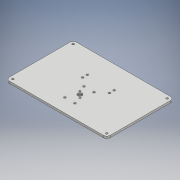
# Autodesk Inventor part: SheetPot
Saved by Autodesk Inventor 2018 (Build 220112000, 112)
## iProperties
Created: 2019-06-03
Part Number: SheetPot
Material: Generic
Document SubType Name: Modeling
Designer: aal_9
Density: 1 g/cm^3
Appearance: Default
Author: aal_9
Autodesk Inventor part; units mm, degrees
ref_plane "YZ Plane" through (0, 0, 0) normal (1, 0, 0) x (0, 1, 0)
ref_plane "XZ Plane" through (0, 0, 0) normal (0, 1, 0) x (-1, 0, 0)
ref_plane "XY Plane" through (0, 0, 0) normal (0, 0, 1) x (1, 0, 0)
sketch "Sketch1" plane through (0, 0, 0) normal (0, 0, 1) x (1, 0, 0)
  line L0 (-75, 65) -> (75, 65)
  line L1 (75, 65) -> (75, -35)
  line L2 (75, -35) -> (-75, -35)
  line L3 (-75, -35) -> (-75, 65)
  point P0 (0, 0)
  dimension "d0" = 150
  dimension "d1" = 100
  dimension "d29" = 65
  dimension "d30" = 75
  constraints: 8 end point, 2 parallel, 1 horizontal, 1 perpendicular
  measures "d0" distance of L0.start L0.end
  measures "d1" distance of L2.end L0.start
  measures "d29" distance from line of point (0, 0) L0
  measures "d30" distance from line of point (0, 0) L3
extrude "Extrusion1" add sketch "Sketch1" along normal blind 3.175
sketch "Sketch2" plane through (0, 0, 0) normal (0, 0, 1) x (1, 0, 0)
  line L0 (75, 65) -> (-75, 65) projected
  line L1 (-75, 65) -> (-75, -35) projected
  line L2 (75, -35) -> (75, 65) projected
  line L3 (-75, -35) -> (75, -35) projected
  point P0 (0, 0)
  point P1 (-70, 60)
  point P2 (70, 60)
  point P3 (70, -30)
  point P4 (-70, -30)
  dimension "d4" = 5
  dimension "d5" = 5
  dimension "d6" = 5
  dimension "d7" = 5
  dimension "d8" = 5
  dimension "d9" = 5
  dimension "d10" = 5
  dimension "d11" = 5
  measures "d4" distance from line of L0 point (-70, 60)
  measures "d5" distance from line of L1 point (-70, 60)
  measures "d6" distance from line of L0 point (70, 60)
  measures "d7" distance from line of L2 point (70, 60)
  measures "d8" distance from line of L3 point (-70, -30)
  measures "d9" distance from line of L1 point (-70, -30)
  measures "d10" distance from line of L2 point (70, -30)
  measures "d11" distance from line of L3 point (70, -30)
hole "Hole1" at (-70, 60, 0) at (70, 60, 0) at (70, -30, 0) at (-70, -30, 0) direction (0, 0, 1) diameter 3 end through all countersink diameter 4 countersink angle 90
fillet "Fillet1" radius 5 4 edges at (-75, 65, 1.5875) (75, 65, 1.5875) (75, -35, 1.5875) (-75, -35, 1.5875)
sketch "Sketch3" plane through (0, 0, 3.175) normal (0, 0, 1) x (1, 0, 0)
  circle A0 centre (0, 0) radius 3.25
  circle A1 centre (4.3841, -4.3841) radius 1.25
  circle A2 centre (-4.3841, 4.3841) radius 1.25
  dimension "d20" = 2.5
  dimension "d21" = 2.5
  dimension "d22" = 6.5
  dimension "d25" = 8.7681
  dimension "d26" = 8.7681
  dimension "d27" = 4.3841
  dimension "d28" = 4.3841
  constraints: 3 centre point, 2 coincident
  measures "d20" diameter of A1
  measures "d21" diameter of A2
  measures "d22" diameter of A0
  measures "d25" horizontal distance of A2.centre A1.centre
  measures "d26" horizontal distance of A1.centre A2.centre
  measures "d27" horizontal distance of point (0, 0) A1.centre
  measures "d28" horizontal distance of point (0, 0) A2.centre
extrude "Extrusion2" cut sketch "Sketch3" against normal up to next
sketch "Sketch4" plane through (0, 0, 0) normal (0, 0, -1) x (-1, 0, 0)
  point P0 (0, 0)
  point P1 (-7.5, 13.5)
  point P2 (7.5, 13.5)
  point P3 (7.5, -15)
  point P4 (-7.5, -15)
  dimension "d33" = 15
  dimension "d34" = 15
  dimension "d35" = 13.5
  dimension "d36" = 15
  dimension "d37" = 7.5
  dimension "d38" = 15
  dimension "d39" = 7.5
  dimension "d40" = 13.5
  measures "d33" distance of point (7.5, 13.5) point (-7.5, 13.5)
  measures "d34" distance of point (7.5, -15) point (-7.5, -15)
  measures "d35" vertical distance of point (0, 0) point (-7.5, 13.5)
  measures "d36" vertical distance of point (-7.5, -15) point (0, 0)
  measures "d37" horizontal distance of point (0, 0) point (-7.5, -15)
  measures "d38" vertical distance of point (7.5, -15) point (0, 0)
  measures "d39" horizontal distance of point (0, 0) point (-7.5, 13.5)
  measures "d40" vertical distance of point (0, 0) point (7.5, 13.5)
hole "Hole2" at (7.5, 13.5, 0) at (-7.5, 13.5, 0) at (-7.5, -15, 0) at (7.5, -15, 0) direction (0, 0, 1) diameter 3 end through all countersink diameter 4 countersink angle 90
sketch "Sketch5" plane through (0, 0, 0) normal (0, 0, -1) x (-1, 0, 0)
  line L0 (70, 65) -> (-70, 65) projected
  line L1 (-75, 60) -> (-75, -30) projected
  line L2 (75, -30) -> (75, 60) projected
  point P0 (0, 0)
  point P1 (-20, 24)
  point P2 (-20, 31)
  point P3 (20, 31)
  point P4 (20, 24)
  dimension "d48" = 0
  dimension "d49" = 0
  dimension "d50" = 34
  dimension "d51" = 34
  dimension "d52" = 7
  dimension "d53" = 7
  dimension "d54" = 55
  dimension "d55" = 55
  measures "d48" horizontal distance of point (-20, 24) point (-20, 31)
  measures "d49" horizontal distance of point (20, 31) point (20, 24)
  measures "d50" distance from line of L0 point (-20, 31)
  measures "d51" distance from line of L0 point (20, 31)
  measures "d52" distance of point (-20, 24) point (-20, 31)
  measures "d53" distance of point (20, 31) point (20, 24)
  measures "d54" distance from line of point (-20, 31) L1
  measures "d55" distance from line of L2 point (20, 31)
hole "Hole3" at (20, 24, 0) at (20, 31, 0) at (-20, 31, 0) at (-20, 24, 0) direction (0, 0, 1) diameter 3 end through all countersink diameter 4 countersink angle 90
equation "\"d37\" = 0.5 * d33"
equation "\"d39\" = 0.5 * d33"
body "Solid1"
